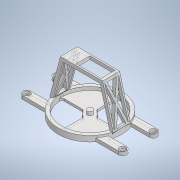
# Autodesk Inventor part: Part1
Saved by Autodesk Inventor 2021 (Build 250183000, 183)
## iProperties
Created: 2025-01-13
Part Number: Part1
Material: Generic
Document SubType Name: Modeling
Designer: 24oscnor
Density: 1 g/cm^3
Appearance: Default
Author: 24oscnor
Autodesk Inventor part; units mm, degrees
ref_plane "YZ Plane" through (0, 0, 0) normal (1, 0, 0) x (0, 1, 0)
ref_plane "XZ Plane" through (0, 0, 0) normal (0, 1, 0) x (-1, 0, 0)
ref_plane "XY Plane" through (0, 0, 0) normal (0, 0, 1) x (1, 0, 0)
sketch "Sketch1" plane through (0, 0, 0) normal (0, 1, 0) x (-1, 0, 0)
  circle A0 centre (0, 0) radius 25
  circle A1 centre (0, 0) radius 28
  circle A2 centre (0, 0) radius 5
  line L0 (5, 0) -> (25, 0)
  line L1 (0, 5) -> (0, 25)
  line L2 (-5, 0) -> (-25, 0)
  line L3 (0, -25) -> (0, -5)
  line L4 (-26.1534, 10) -> (-42.2486, 10)
  line L5 (-42.2486, 10) -> (-42.2486, 17)
  line L6 (-42.2486, 17) -> (-22.2486, 17)
  line L7 (-26.1534, -10) -> (-42.2486, -10)
  line L8 (-42.2486, -10) -> (-42.2486, -17)
  line L9 (-42.2486, -17) -> (-22.2486, -17)
  line L10 (26.1534, 10) -> (42.2486, 10)
  line L11 (42.2486, 10) -> (42.2486, 17)
  line L12 (42.2486, 17) -> (22.2486, 17)
  line L13 (22.2486, -17) -> (42.2486, -17)
  line L14 (42.2486, -17) -> (42.2486, -10)
  line L15 (42.2486, -10) -> (26.1534, -10)
  circle A3 centre (-42.2486, 13.5) radius 3.5
  circle A4 centre (-42.2486, -13.5) radius 3.5
  circle A5 centre (42.2486, -13.5) radius 3.5
  circle A6 centre (42.2486, 13.5) radius 3.5
  point P0 (-42.2486, 17)
  point P1 (-42.2486, -10)
  point P2 (42.2486, -10)
  dimension "d0" = 50
  dimension "d1" = 3
  dimension "d6" = 10
  dimension "d7" = 20
  dimension "d8" = 20
  dimension "d9" = 20
  dimension "d10" = 90
  dimension "d15" = 7
  dimension "d16" = 7
  dimension "d17" = 20
  dimension "d18" = 20
  dimension "d19" = 10
  dimension "d20" = 10
  constraints: 32 end point, 14 point on line, 8 point on circle, 5 perpendicular, 4 midpoint, 3 coincident, 2 centre point, 1 horizontal, 1 parallel, 22 other
  measures "d0" diameter of A0
  measures "d6" diameter of A2
  measures "d7" distance of L2.start L2.end
  measures "d8" distance of L3.start L3.end
  measures "d9" distance of L0.start L0.end
  measures "d10" angle of L2 L1
  measures "d15" distance of L4.end L5.end
  measures "d16" distance of L7.end L8.end
  measures "d17" distance of L5.end L6.end
  measures "d18" distance of L11.end L12.end
  measures "d19" distance from line of point (0, 0) L4
  measures "d20" distance from line of point (0, 0) L7
extrude "Extrusion1" add sketch "Sketch1" along normal blind 2 contours A0 L3 A2 L0 | L1 A2 L2 A0 | A2
extrude "Extrusion2" add sketch "Sketch1" along normal blind 5 contours A1
fillet "Fillet1" radius 2 8 edges at (0, 1, 5) (-5, 1, 0) (5, 1, 0) (0, 1, -5) (0, 1, -25) (25, 1, 0) (-25, 1, 0) (0, 1, 25)
sketch "Sketch2" plane through (0, 2, 0) normal (0, 1, 0) x (1, 0, 0)
  circle A0 centre (0, 0) radius 2.5
  dimension "d12" = 5
  constraints: 1 centre point, 1 coincident
  measures "d12" diameter of A0
extrude "Extrusion3" add sketch "Sketch2" along normal blind 3
extrude "Extrusion4" add sketch "Sketch1" along normal blind 3 contours A1 L12 A6 L10 | L15 A5 L13 A1 | A6 L11 | L11 A6 | A5 L14 | L14 A5 | A1 L4 A3 L6 | L9 A4 L7 A1 | A3 L5 | L5 A3 | A4 L8 | L8 A4
sketch "Sketch3" plane through (0, 3, 0) normal (0, 1, 0) x (1, 0, 0)
  circle A0 centre (42.2486, 13.5) radius 2.75
  arc A1 (42.2486, 10) -> (42.2486, 17) centre (42.2486, 13.5) ccw projected
  line L0 (0, -49.0118) -> (0, 57.5939) construction
  line L1 (54.3673, 0) -> (-51.4136, 0) construction
  circle A2 centre (42.2486, -13.5) radius 2.75
  circle A3 centre (-42.2486, 13.5) radius 2.75
  circle A4 centre (-42.2486, -13.5) radius 2.75
  circle A5 centre (42.2486, 13.5) radius 1.625
  circle A6 centre (42.2486, -13.5) radius 1.625
  circle A7 centre (-42.2486, 13.5) radius 1.625
  circle A8 centre (-42.2486, -13.5) radius 1.625
  point P0 (0, 0)
  dimension "d23" = 5.5
  dimension "d24" = 0
  dimension "d25" = 0
  dimension "d28" = 3.25
  constraints: 8 centre point, 6 symmetric about line, 4 end point, 1 coincident, 1 horizontal, 1 vertical, 6 other
  measures "d23" diameter of A0
  measures "d24" distance of A1.centre A0.centre
  measures "d25" distance of A1.centre A0.centre
  measures "d28" diameter of A5
extrude "Extrusion5" cut sketch "Sketch3" against normal blind 2 contours A0 | A2 | A3 | A4 | A5 | A6 | A7 | A8
extrude "Extrusion6" cut sketch "Sketch3" against normal through all contours A5 | A6 | A7 | A8
sketch "Sketch4" plane through (0, 0, 0) normal (0, 0, 1) x (1, 0, 0)
  line L0 (28, 5) -> (-28, 5) projected
  line L1 (-28, 5) -> (-18.6218, 40)
  line L2 (-18.6218, 40) -> (-15.6218, 40)
  line L3 (-25, 5) -> (25, 5) projected
  line L4 (-15.6218, 40) -> (-25, 5)
  line L5 (-25, 5) -> (-28, 5)
  line L6 (0, 37.1698) -> (0, -14.7321) construction
  line L7 (28, 5) -> (18.6218, 40)
  line L8 (18.6218, 40) -> (-15.6218, 40)
  line L9 (25, 5) -> (15.6218, 40)
  line L10 (-16.4256, 37) -> (16.4256, 37)
  point P0 (0, 0)
  dimension "d31" = 75
  dimension "d32" = 35
  dimension "d34" = 75
  dimension "d36" = 3
  constraints: 18 end point, 3 parallel, 3 point on line, 1 collinear, 1 horizontal, 1 symmetric about line, 1 vertical
  measures "d31" angle of L0 L4
  measures "d32" distance between parallel lines of L3 L2
  measures "d34" angle of L0 L7
  measures "d36" distance between parallel lines of L8 L10
extrude "Extrusion7" add sketch "Sketch4" along normal mid plane 15 contours L0 L9 L8 L7 | L0 L1 L2 L4 | L10 L4 L8 L9
sketch "Sketch5" plane through (0, 0, -7.5) normal (0, 0, -1) x (-1, 0, 0)
  line L0 (-26.9768, 5) -> (-28, 5) projected
  line L1 (-24.9053, 2) -> (-24.9053, 0) projected
  line L2 (-28, 5) -> (-24.9053, 0)
  line L3 (26.9768, 5) -> (28, 5) projected
  line L4 (24.9053, 2) -> (24.9053, 0) projected
  line L5 (28, 5) -> (24.9053, 0)
  line L6 (24.9053, 0) -> (25, 5)
  line L7 (25, 5) -> (25, 2) projected
  line L8 (28, 5) -> (-28, 5)
  line L9 (-28, 0) -> (-28, 5) projected
  line L10 (26.9768, 5) -> (-26.9768, 5) projected
  line L11 (-25.0099, 5) -> (-24.9053, 0)
  point P0 (0, 0)
  constraints: 10 end point, 2 point on line, 1 perpendicular
extrude "Extrusion8" add sketch "Sketch5" against normal blind 15
sketch "Sketch7" plane through (-18.6218, 40, 7.5) normal (0, 1, 0) x (1, 0, 0)
  line L0 (12.3218, 1.3) -> (34.6718, 1.3)
  line L1 (34.6718, 1.3) -> (34.6718, 13.7)
  line L2 (34.6718, 13.7) -> (12.3218, 13.7)
  line L3 (12.3218, 13.7) -> (12.3218, 1.3)
  line L4 (37.2436, 0) -> (0, 0) projected
  point P0 (18.6218, 7.5)
  dimension "d46" = 22.35
  dimension "d47" = 12.4
  dimension "d48" = 1.3
  dimension "d49" = 16.05
  constraints: 8 end point, 2 parallel, 1 horizontal, 1 perpendicular
  measures "d46" distance of L0.start L0.end
  measures "d47" distance of L0.end L1.end
  measures "d48" distance between parallel lines of L4 L0
  measures "d49" distance from line of point (18.622, 7.5) L1
extrude "Extrusion9" cut sketch "Sketch7" against normal blind 10
sketch "Sketch8" plane through (18.6218, 40, 7.5) normal (0.9659258, 0.258819, 0) x (0, 0, -1)
  line L0 (15, -2.3294) -> (0, -2.3294) projected
  line L1 (1.3, -34.9347) -> (13.7, -34.9347)
  line L2 (13.7, -34.9347) -> (13.7, -2.3294)
  line L3 (13.7, -2.3294) -> (1.3, -2.3294)
  line L4 (1.3, -2.3294) -> (1.3, -34.9347)
  line L5 (0, -36.2347) -> (0, 0) projected
  line L6 (15, 0) -> (15, -36.2347) projected
  line L7 (7.5, -36.2347) -> (0, -36.2347) projected
  point P0 (7.5, -33.8174)
  point P1 (1.3, -2.3294)
  dimension "d52" = 1.3
  dimension "d53" = 1.3
  dimension "d54" = 1.3
  constraints: 8 end point, 2 parallel, 1 horizontal, 1 perpendicular, 1 point on line
  measures "d52" distance between parallel lines of L5 L4
  measures "d53" distance between parallel lines of L6 L2
  measures "d54" distance between parallel lines of L7 L1
extrude "Extrusion10" cut sketch "Sketch8" against normal up to next
sketch "Sketch9" plane through (-18.6218, 40, -7.5) normal (-0.9659258, 0.258819, 0) x (0, 0, 1)
  line L0 (0, -2.3294) -> (15, -2.3294) projected
  line L1 (1.3, -2.3294) -> (13.7, -2.3294)
  line L2 (13.7, -2.3294) -> (13.7, -34.9347)
  line L3 (13.7, -34.9347) -> (1.3, -34.9347)
  line L4 (1.3, -34.9347) -> (1.3, -2.3294)
  line L5 (7.5, -36.2347) -> (15, -36.2347) projected
  line L6 (0, -36.2347) -> (0, 0) projected
  line L7 (15, 0) -> (15, -36.2347) projected
  point P0 (7.5, -33.8174)
  point P1 (13.7, -2.3294)
  dimension "d57" = 1.3
  dimension "d58" = 1.3
  dimension "d59" = 1.3
  constraints: 8 end point, 2 parallel, 1 horizontal, 1 perpendicular, 1 point on line
  measures "d57" distance between parallel lines of L3 L5
  measures "d58" distance between parallel lines of L6 L4
  measures "d59" distance between parallel lines of L7 L2
extrude "Extrusion11" cut sketch "Sketch9" against normal up to surface (2.8978 mm away)
sketch "Sketch10" plane through (-18.6218, 40, -7.5) normal (-0.9659258, 0.258819, 0) x (0, 0, 1)
  line L0 (1.3, -2.3294) -> (1.3, -34.9347) projected
  line L1 (1.3, -34.9347) -> (11.6025, -2.3294)
  line L2 (1.3, -2.3294) -> (13.7, -2.3294) projected
  line L3 (13.7, -20.615) -> (13.7, 7.622) projected
  line L4 (13.7, -2.3294) -> (3.3975, -34.9347)
  line L5 (13.7, -34.9347) -> (1.3, -34.9347) projected
  line L6 (1.3, 7.622) -> (1.3, -20.615) projected
  line L7 (13.7, -2.3294) -> (13.7, -34.9347) projected
  line L8 (7.5, -34.9347) -> (7.5, -2.3294) construction
  line L9 (13.7, -34.9347) -> (3.3975, -2.3294)
  line L10 (1.3, -2.3294) -> (11.6025, -34.9347)
  point P0 (7.5, -33.8174)
  point P1 (6.4513, -18.632)
  point P2 (7.5, -21.951)
  point P3 (8.5487, -18.632)
  point P4 (7.5, -15.313)
  point P5 (3.3975, -2.3294)
  dimension "d62" = 2
  dimension "d64" = 35.071
  constraints: 10 end point, 3 point on line, 3 symmetric about line, 2 midpoint, 1 parallel
  measures "d62" distance between parallel lines of L1 L4
  measures "d64" angle of L9 L4
extrude "Extrusion12" add sketch "Sketch10" against normal blind 3 contours L2 L9 L1 L10 | L10 L4 L5 L1 | L1 L9 L4 L10 | L2 L4 L9 L1 | L4 L9 L5 L10
sketch "Sketch11" plane through (18.6218, 40, 7.5) normal (0.9659258, 0.258819, 0) x (0, 0, -1)
  line L0 (13.7, -34.9347) -> (1.3, -34.9347) projected
  line L1 (13.7, -34.9347) -> (3.3975, -2.3294)
  line L2 (13.7, -2.3294) -> (1.3, -2.3294) projected
  line L3 (1.3, -22.0639) -> (1.3, 6.1732) projected
  line L4 (1.3, -34.9347) -> (1.3, -2.3294) projected
  line L5 (1.3, -2.3294) -> (11.6025, -34.9347)
  line L6 (7.5, -2.3294) -> (7.5, -34.9347) construction
  line L7 (1.3, -34.9347) -> (11.6025, -2.3294)
  line L8 (13.7, -2.3294) -> (3.3975, -34.9347)
  point P0 (7.5, -33.8174)
  point P1 (7.5, -21.951)
  point P2 (8.5487, -18.632)
  point P3 (11.6025, -2.3294)
  point P4 (7.5, -15.313)
  point P5 (6.4513, -18.632)
  dimension "d68" = 2
  constraints: 10 end point, 2 midpoint, 2 point on line, 2 symmetric about line, 1 parallel
  measures "d68" distance between parallel lines of L5 L1
extrude "Extrusion13" add sketch "Sketch11" against normal blind 3 contours L0 L5 L8 L1 | L8 L5 L7 L1 | L1 L7 L2 L8 | L0 L7 L5 L8 | L7 L5 L2 L1
body "Solid1"
